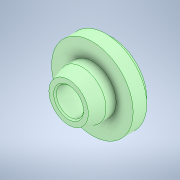
# Autodesk Inventor part: EncoderCodeWheelMount HTD-3M
Saved by Autodesk Inventor 2022.2 (Build 262287000, 287)
## iProperties
Created: 2019-07-04
Part Number: EncoderCodeWheelMount HTD-3M
Material: Generic
Document SubType Name: Modeling
Designer: Jochen
Density: 1 g/cm^3
Appearance: Default
Sending System: SolidWorks 2017
Last Author: Felix
Last Saved: 2021-02-23
Author: Jochen
Autodesk Inventor part; units mm, degrees
ref_plane "YZ Plane" through (0, 0, 0) normal (1, 0, 0) x (0, 1, 0)
ref_plane "XZ Plane" through (0, 0, 0) normal (0, 1, 0) x (-1, 0, 0)
ref_plane "XY Plane" through (0, 0, 0) normal (0, 0, 1) x (1, 0, 0)
sketch "Sketch2" plane through (0, 0, 0) normal (0, 0, 1) x (1, 0, 0)
  arc A0 (4.6801, -5.9941) -> (3.9272, -6.6466) centre (4.8647, -6.9678) ccw
  line L0 (4.7371, -5.9833) -> (4.6801, -5.9941)
  arc A1 (5.6766, -6.315) -> (4.7371, -5.9833) centre (4.9216, -6.957) ccw
  line L1 (5.9882, -6.6814) -> (5.6766, -6.315)
  arc A2 (5.9882, -6.6814) -> (6.2072, -6.726) centre (6.1261, -6.5642) ccw
  arc A3 (6.2072, -6.726) -> (6.2757, -6.691) centre (4.0234, -2.3731) ccw
  arc A4 (6.2757, -6.691) -> (6.3677, -6.4873) centre (6.1919, -6.5305) ccw
  line L2 (6.2529, -6.0202) -> (6.3677, -6.4873)
  arc A5 (6.5336, -5.0642) -> (6.2529, -6.0202) centre (7.2152, -5.7836) ccw
  arc A6 (1.0024, -4.4747) -> (0.0961, -4.0608) centre (0.1934, -5.0471) ccw
  arc A7 (-0.5711, -3.9879) -> (-0.3826, -4.1081) centre (-0.4003, -3.9279) ccw
  arc A8 (-0.596, -3.9153) -> (-0.5711, -3.9879) centre (4.0234, -2.3731) ccw
  arc A9 (-0.5208, -3.7048) -> (-0.596, -3.9153) centre (-0.4243, -3.8579) ccw
  line L3 (-0.5208, -3.7048) -> (-0.1137, -3.4485)
  line L4 (0.3483, -2.5658) -> (0.3457, -2.5078)
  arc A10 (-0.1137, -3.4485) -> (0.3483, -2.5658) centre (-0.6417, -2.6099) ccw
  arc A11 (0.3457, -2.5078) -> (-0.1929, -1.6697) centre (-0.6443, -2.5519) ccw
  line L5 (0.0961, -4.0608) -> (-0.3826, -4.1081)
  line L6 (0.8567, 0.4982) -> (0.6149, 0.914)
  arc A12 (0.8567, -0.4982) -> (0.8567, 0.4982) centre (0, 0) ccw
  line L7 (0.8275, -0.5483) -> (0.8567, -0.4982)
  arc A13 (-0.0384, -1.0411) -> (0.8275, -0.5483) centre (-0.0292, -0.0501) ccw
  line L8 (-0.5193, -1.0366) -> (-0.0384, -1.0411)
  arc A14 (-0.5193, -1.0366) -> (-0.6964, -1.173) centre (-0.521, -1.2176) ccw
  arc A15 (-0.6964, -1.173) -> (-0.7148, -1.2476) centre (4.0234, -2.3731) ccw
  line L9 (-0.1929, -1.6697) -> (-0.6211, -1.4506)
  arc A16 (-0.7148, -1.2476) -> (-0.6211, -1.4506) centre (-0.5387, -1.2895) ccw
  arc A17 (0.6458, 1.1354) -> (0.6149, 0.914) centre (0.7714, 1.005) ccw
  arc A18 (0.7016, 1.1882) -> (0.6458, 1.1354) centre (4.0234, -2.3731) ccw
  arc A19 (0.9243, 1.2072) -> (0.7016, 1.1882) centre (0.8251, 1.0558) ccw
  line L10 (0.9243, 1.2072) -> (1.3266, 0.9434)
  arc A20 (1.3266, 0.9434) -> (2.3214, 0.8898) centre (1.87, 1.7721) ccw
  line L11 (2.3214, 0.8898) -> (2.3731, 0.9162)
  arc A21 (2.3731, 0.9162) -> (2.9117, 1.7544) centre (1.9217, 1.7985) ccw
  line L12 (2.9117, 1.7544) -> (2.9331, 2.2349)
  arc A22 (3.0788, 2.4044) -> (2.9331, 2.2349) centre (3.1139, 2.2269) ccw
  arc A23 (3.1543, 2.4187) -> (3.0788, 2.4044) centre (4.0234, -2.3731) ccw
  arc A24 (3.5477, 1.8749) -> (4.3557, 1.292) centre (4.4529, 2.2782) ccw
  line L13 (3.3519, 2.3143) -> (3.5477, 1.8749)
  arc A25 (3.3519, 2.3143) -> (3.1543, 2.4187) centre (3.1866, 2.2406) ccw
  line L14 (4.3557, 1.292) -> (4.4134, 1.2863)
  arc A26 (4.4134, 1.2863) -> (5.3197, 1.7002) centre (4.5106, 2.2725) ccw
  line L15 (5.3197, 1.7002) -> (5.5975, 2.0929)
  arc A27 (5.8117, 2.1567) -> (5.5975, 2.0929) centre (5.7452, 1.9883) ccw
  arc A28 (5.8829, 2.1279) -> (5.8117, 2.1567) centre (4.0234, -2.3731) ccw
  arc A29 (5.9927, 1.9332) -> (5.8829, 2.1279) centre (5.8138, 1.9606) ccw
  line L16 (5.9927, 1.9332) -> (5.9199, 1.4577)
  arc A30 (5.9199, 1.4577) -> (6.2844, 0.5305) centre (6.8994, 1.3076) ccw
  line L17 (6.2844, 0.5305) -> (6.3299, 0.4945)
  arc A31 (6.3299, 0.4945) -> (7.3161, 0.3527) centre (6.9449, 1.2716) ccw
  line L18 (7.3161, 0.3527) -> (7.7621, 0.5329)
  arc A32 (7.9768, 0.4708) -> (7.7621, 0.5329) centre (7.8298, 0.3651) ccw
  arc A33 (8.0212, 0.408) -> (7.9768, 0.4708) centre (4.0234, -2.3731) ccw
  arc A34 (8.0083, 0.1849) -> (8.0212, 0.408) centre (7.8726, 0.3047) ccw
  line L19 (8.0083, 0.1849) -> (7.6899, -0.1757)
  arc A35 (7.6899, -0.1757) -> (7.4953, -1.1528) centre (8.4328, -0.8316) ccw
  line L20 (7.4953, -1.1528) -> (7.5141, -1.2077)
  arc A36 (7.5141, -1.2077) -> (8.2671, -1.8601) centre (8.4516, -0.8865) ccw
  line L21 (8.2671, -1.8601) -> (8.7396, -1.9497)
  arc A37 (8.8867, -2.1181) -> (8.7396, -1.9497) centre (8.7059, -2.1275) ccw
  arc A38 (8.8901, -2.1948) -> (8.8867, -2.1181) centre (4.0234, -2.3731) ccw
  line L22 (8.7586, -2.3756) -> (8.2958, -2.5068)
  arc A39 (8.7586, -2.3756) -> (8.8901, -2.1948) centre (8.7092, -2.2014) ccw
  arc A40 (8.2958, -2.5068) -> (7.6039, -3.2236) centre (8.5662, -3.4602) ccw
  line L23 (7.6039, -3.2236) -> (7.59, -3.2799)
  arc A41 (7.59, -3.2799) -> (7.8707, -4.2359) centre (8.5523, -3.5165) ccw
  line L24 (7.8707, -4.2359) -> (8.2199, -4.5667)
  arc A42 (8.2525, -4.7879) -> (8.2199, -4.5667) centre (8.0954, -4.6981) ccw
  arc A43 (8.2139, -4.8543) -> (8.2525, -4.7879) centre (4.0234, -2.3731) ccw
  arc A44 (8.0056, -4.9352) -> (8.2139, -4.8543) centre (8.0582, -4.7621) ccw
  line L25 (8.0056, -4.9352) -> (7.5453, -4.7954)
  arc A45 (7.5453, -4.7954) -> (6.5757, -5.0243) centre (7.2573, -5.7437) ccw
  line L26 (6.5757, -5.0243) -> (6.5336, -5.0642)
  line L27 (3.9272, -6.6466) -> (3.7713, -7.1016)
  arc A46 (3.5837, -7.2232) -> (3.7713, -7.1016) centre (3.6, -7.0429) ccw
  arc A47 (3.5072, -7.2157) -> (3.5837, -7.2232) centre (4.0234, -2.3731) ccw
  line L28 (3.347, -7.0598) -> (3.283, -6.583)
  arc A48 (3.347, -7.0598) -> (3.5072, -7.2157) centre (3.5264, -7.0357) ccw
  line L29 (1.0359, -4.5221) -> (1.0024, -4.4747)
  arc A49 (1.1244, -5.5144) -> (1.0359, -4.5221) centre (0.2269, -5.0944) ccw
  line L30 (0.9206, -5.9501) -> (1.1244, -5.5144)
  arc A50 (0.9206, -5.9501) -> (0.9711, -6.1679) centre (1.0845, -6.0268) ccw
  arc A51 (0.9711, -6.1679) -> (1.0313, -6.2155) centre (4.0234, -2.3731) ccw
  arc A52 (1.0313, -6.2155) -> (1.2548, -6.2147) centre (1.1425, -6.0727) ccw
  line L31 (1.632, -5.9162) -> (1.2548, -6.2147)
  line L32 (2.672, -5.7961) -> (2.6182, -5.7744)
  arc A53 (2.6182, -5.7744) -> (1.632, -5.9162) centre (2.247, -6.6932) ccw
  arc A54 (3.283, -6.583) -> (2.672, -5.7961) centre (2.3008, -6.715) ccw
  circle A55 centre (4.0234, -2.3731) radius 2
  circle A56 centre (4.0234, -2.3731) radius 6
  circle A57 centre (4.0234, -2.3731) radius 3.5
  arc A58 (0.9433, -5.4297) -> (0.8726, -4.6376) centre (0.2269, -5.0944) ccw
  line L33 (0.9433, -5.4297) -> (0.7394, -5.8653)
  arc A59 (0.7394, -5.8653) -> (0.8457, -6.3237) centre (1.0845, -6.0268) ccw
  arc A60 (0.8457, -6.3237) -> (0.9084, -6.3733) centre (4.0234, -2.3731) ccw
  arc A61 (0.9084, -6.3733) -> (1.379, -6.3715) centre (1.1425, -6.0727) ccw
  line L34 (1.379, -6.3715) -> (1.7561, -6.073)
  arc A62 (2.5433, -5.9598) -> (1.7561, -6.073) centre (2.247, -6.6932) ccw
  line L35 (2.5433, -5.9598) -> (2.5971, -5.9815)
  arc A63 (3.0848, -6.6097) -> (2.5971, -5.9815) centre (2.3008, -6.715) ccw
  line L36 (3.0848, -6.6097) -> (3.1488, -7.0864)
  arc A64 (3.1488, -7.0864) -> (3.486, -7.4145) centre (3.5264, -7.0357) ccw
  arc A65 (3.486, -7.4145) -> (3.5656, -7.4224) centre (4.0234, -2.3731) ccw
  arc A66 (3.5656, -7.4224) -> (3.9605, -7.1664) centre (3.6, -7.0429) ccw
  line L37 (3.9605, -7.1664) -> (4.1164, -6.7114)
  arc A67 (4.7174, -6.1906) -> (4.1164, -6.7114) centre (4.8647, -6.9678) ccw
  line L38 (4.7174, -6.1906) -> (4.7744, -6.1798)
  arc A68 (5.5242, -6.4446) -> (4.7744, -6.1798) centre (4.9216, -6.957) ccw
  line L39 (5.5242, -6.4446) -> (5.8358, -6.811)
  arc A69 (5.8358, -6.811) -> (6.2969, -6.9047) centre (6.1261, -6.5642) ccw
  arc A70 (6.2969, -6.9047) -> (6.3681, -6.8683) centre (4.0234, -2.3731) ccw
  arc A71 (6.3681, -6.8683) -> (6.5619, -6.4395) centre (6.1919, -6.5305) ccw
  line L40 (6.5619, -6.4395) -> (6.4471, -5.9724)
  arc A72 (6.6711, -5.2094) -> (6.4471, -5.9724) centre (7.2152, -5.7836) ccw
  line L41 (6.6711, -5.2094) -> (6.7132, -5.1695)
  arc A73 (7.4872, -4.9868) -> (6.7132, -5.1695) centre (7.2573, -5.7437) ccw
  line L42 (7.4872, -4.9868) -> (7.9474, -5.1266)
  arc A74 (7.9474, -5.1266) -> (8.386, -4.9562) centre (8.0582, -4.7621) ccw
  arc A75 (8.386, -4.9562) -> (8.4262, -4.887) centre (4.0234, -2.3731) ccw
  arc A76 (8.4262, -4.887) -> (8.3574, -4.4215) centre (8.0954, -4.6981) ccw
  line L43 (8.3574, -4.4215) -> (8.0083, -4.0907)
  arc A77 (7.7842, -3.3277) -> (8.0083, -4.0907) centre (8.5523, -3.5165) ccw
  line L44 (7.7842, -3.3277) -> (7.7981, -3.2713)
  arc A78 (8.3504, -2.6992) -> (7.7981, -3.2713) centre (8.5662, -3.4602) ccw
  line L45 (8.3504, -2.6992) -> (8.8132, -2.568)
  arc A79 (8.8132, -2.568) -> (9.09, -2.1875) centre (8.7092, -2.2014) ccw
  arc A80 (9.09, -2.1875) -> (9.0864, -2.1076) centre (4.0234, -2.3731) ccw
  arc A81 (9.0864, -2.1076) -> (8.7769, -1.7532) centre (8.7059, -2.1275) ccw
  line L46 (8.7769, -1.7532) -> (8.3043, -1.6636)
  arc A82 (7.7033, -1.1429) -> (8.3043, -1.6636) centre (8.4516, -0.8865) ccw
  line L47 (7.7033, -1.1429) -> (7.6845, -1.088)
  arc A83 (7.8398, -0.3081) -> (7.6845, -1.088) centre (8.4328, -0.8316) ccw
  line L48 (7.8398, -0.3081) -> (8.1582, 0.0525)
  arc A84 (8.1582, 0.0525) -> (8.1853, 0.5223) centre (7.8726, 0.3047) ccw
  arc A85 (8.1853, 0.5223) -> (8.1391, 0.5876) centre (4.0234, -2.3731) ccw
  arc A86 (8.1391, 0.5876) -> (7.6871, 0.7183) centre (7.8298, 0.3651) ccw
  line L49 (7.6871, 0.7183) -> (7.2412, 0.5382)
  arc A87 (6.454, 0.6514) -> (7.2412, 0.5382) centre (6.9449, 1.2716) ccw
  line L50 (6.454, 0.6514) -> (6.4085, 0.6874)
  arc A88 (6.1175, 1.4274) -> (6.4085, 0.6874) centre (6.8994, 1.3076) ccw
  line L51 (6.1175, 1.4274) -> (6.1904, 1.9029)
  arc A89 (6.1904, 1.9029) -> (5.9593, 2.3128) centre (5.8138, 1.9606) ccw
  arc A90 (5.9593, 2.3128) -> (5.8851, 2.3427) centre (4.0234, -2.3731) ccw
  arc A91 (5.8851, 2.3427) -> (5.4342, 2.2084) centre (5.7452, 1.9883) ccw
  line L52 (5.4342, 2.2084) -> (5.1564, 1.8157)
  arc A92 (4.433, 1.4853) -> (5.1564, 1.8157) centre (4.5106, 2.2725) ccw
  line L53 (4.433, 1.4853) -> (4.3753, 1.491)
  arc A93 (3.7304, 1.9563) -> (4.3753, 1.491) centre (4.4529, 2.2782) ccw
  line L54 (3.7304, 1.9563) -> (3.5346, 2.3957)
  arc A94 (3.5346, 2.3957) -> (3.1186, 2.6155) centre (3.1866, 2.2406) ccw
  arc A95 (3.1186, 2.6155) -> (3.04, 2.6006) centre (4.0234, -2.3731) ccw
  arc A96 (3.04, 2.6006) -> (2.7333, 2.2438) centre (3.1139, 2.2269) ccw
  line L55 (2.7333, 2.2438) -> (2.7119, 1.7633)
  arc A97 (2.282, 1.0943) -> (2.7119, 1.7633) centre (1.9217, 1.7985) ccw
  line L56 (2.282, 1.0943) -> (2.2303, 1.0679)
  arc A98 (1.4362, 1.1106) -> (2.2303, 1.0679) centre (1.87, 1.7721) ccw
  line L57 (1.4362, 1.1106) -> (1.034, 1.3744)
  arc A99 (1.034, 1.3744) -> (0.5652, 1.3345) centre (0.8251, 1.0558) ccw
  arc A100 (0.5652, 1.3345) -> (0.5071, 1.2794) centre (4.0234, -2.3731) ccw
  arc A101 (0.5071, 1.2794) -> (0.442, 0.8134) centre (0.7714, 1.005) ccw
  line L58 (0.442, 0.8134) -> (0.6838, 0.3976)
  arc A102 (0.6838, -0.3976) -> (0.6838, 0.3976) centre (0, 0) ccw
  line L59 (0.6838, -0.3976) -> (0.6546, -0.4478)
  arc A103 (-0.0365, -0.8411) -> (0.6546, -0.4478) centre (-0.0292, -0.0501) ccw
  line L60 (-0.0365, -0.8411) -> (-0.5175, -0.8366)
  arc A104 (-0.5175, -0.8366) -> (-0.8903, -1.1237) centre (-0.521, -1.2176) ccw
  arc A105 (-0.8903, -1.1237) -> (-0.9094, -1.2014) centre (4.0234, -2.3731) ccw
  arc A106 (-0.9094, -1.2014) -> (-0.7122, -1.6286) centre (-0.5387, -1.2895) ccw
  line L61 (-0.7122, -1.6286) -> (-0.284, -1.8477)
  arc A107 (0.1459, -2.5167) -> (-0.284, -1.8477) centre (-0.6443, -2.5519) ccw
  line L62 (0.1459, -2.5167) -> (0.1485, -2.5747)
  arc A108 (-0.2203, -3.2792) -> (0.1485, -2.5747) centre (-0.6417, -2.6099) ccw
  line L63 (-0.2203, -3.2792) -> (-0.6273, -3.5355)
  arc A109 (-0.6273, -3.5355) -> (-0.7857, -3.9786) centre (-0.4243, -3.8579) ccw
  arc A110 (-0.7857, -3.9786) -> (-0.7598, -4.0543) centre (4.0234, -2.3731) ccw
  arc A111 (-0.7598, -4.0543) -> (-0.3629, -4.3071) centre (-0.4003, -3.9279) ccw
  line L64 (-0.3629, -4.3071) -> (0.1157, -4.2599)
  arc A112 (0.8391, -4.5902) -> (0.1157, -4.2599) centre (0.1934, -5.0471) ccw
  line L65 (0.8391, -4.5902) -> (0.8726, -4.6376)
  point P0 (4.0234, -2.3731)
  dimension "d35" = 4
  dimension "d36" = 12
  dimension "d37" = 7
  dimension "d45" = 0.2
  constraints: 220 point on circle, 132 end point, 113 centre point, 3 coincident, 87 other
  measures "d35" diameter of A55
  measures "d36" diameter of A56
  measures "d37" diameter of A57
  measures "d45" radial gap between concentric circles of A49 A58
extrude "Extrusion5" add sketch "Sketch2" along normal blind 0.8 contours A56
chamfer "Chamfer5" distance 0.8 angle 45 1 edges at (-1.9766, -2.3731, 0)
extrude "Extrusion7" add sketch "Sketch2" along normal blind 2 from surface at 0.8 contours A0 L27 A46 A47 A48 L28 A54 L32 A53 L31 A52 A51 A50 L30 A49 L29 A6 L5 A7 A8 A9 L3 A10 L4 A11 L9 A16 A15 A14 L8 A13 L7 A12 L6 A17 A18 A19 L10 A20 L11 A21 L12 A22 A23 A25 L13 A24 L14 A26 L15 A27 A28 A29 L16 A30 L17 A31 L18 A32 A33 A34 L19 A35 L20 A36 L21 A37 A38 A39 L22 A40 L23 A41 L24 A42 A43 A44 L25 A45 L26 A5 L2 A4 A3 A2 L1 A1 L0 | A56 | A57 | A58 L65 A112 L64 A111 A110 A109 L63 A108 L62 A107 L61 A106 A105 A104 L60 A103 L59 A102 L58 A101 A100 A99 L57 A98 L56 A97 L55 A96 A95 A94 L54 A93 L53 A92 L52 A91 A90 A89 L51 A88 L50 A87 L49 A86 A85 A84 L48 A83 L47 A82 L46 A81 A80 A79 L45 A78 L44 A77 L43 A76 A75 A74 L42 A73 L41 A72 L40 A71 A70 A69 L39 A68 L38 A67 L37 A66 A65 A64 L36 A63 L35 A62 L34 A61 A60 A59 L33
extrude "Extrusion8" add sketch "Sketch2" along normal blind 3.5 from surface at 2.8 contours A57
chamfer "Chamfer6" distance 0.2 angle 45 2 edges at (2.0234, -2.3731, 0.8) (2.0234, -2.3731, 6.3)
chamfer "Chamfer7" distance 2 distance2 0.6 1 edges at (0.5234, -2.3731, 6.3) measured on face at (0.5234, -2.3731, 5.8)
body "Solid1"
body "Solid5"
body "Solid6"
